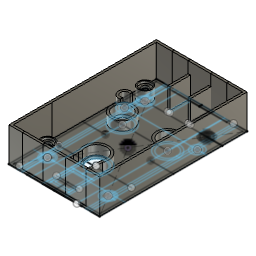
White_body v4 (Autodesk Fusion 360 design; units mm, degrees)
Autodesk Fusion 360 part; units mm, degrees
sketch "Sketch1" plane through (0, 0, 0) normal (0, 0, 1) x (1, 0, 0)
  line L0 (20, 32.5) -> (-20, 32.5)
  line L1 (-20, 32.5) -> (-20, -32.5)
  line L2 (-20, -32.5) -> (20, -32.5)
  line L3 (20, -32.5) -> (20, 32.5)
  line L4 (20, 32.5) -> (-20, -32.5) construction
  line L5 (-20, 32.5) -> (20, -32.5) construction
  line L6 (0, -32.5) -> (-5, -32.5)
  line L7 (-5, -32.5) -> (5, -32.5)
  line L8 (5, -32.5) -> (5, -16.2913)
  line L9 (-3.9274, -31.5) -> (4, -31.5)
  line L10 (-4, -17.7749) -> (-3.9274, -31.5)
  line L11 (4, -31.5) -> (4, -17.7749)
  line L12 (-5, -32.5) -> (-5, -16.2913)
  line L13 (-5, -16.2913) -> (-5, -32.5)
  line L14 (0, -31.5) -> (0, -32.5)
  circle A0 centre (0, -14) radius 4
  line L15 (4, -17.7749) -> (4, -16.0616)
  line L16 (19, -31.5) -> (19, 31.5)
  line L17 (19, 31.5) -> (-19, 31.5)
  line L18 (-19, 31.5) -> (-19, -31.5)
  line L19 (-19, -31.5) -> (19, -31.5)
  line L20 (-4, -17.7749) -> (-4, -16.0616)
  arc A1 (5, -16.2913) -> (-5, -16.2913) centre (0, -14) ccw
  arc A2 (4, -16.0616) -> (-4, -16.0616) centre (0, -14) ccw
  line L21 (-19, -30.875) -> (-17, -30.875)
  line L22 (-20, 32.5) -> (-14, 32.5)
  line L23 (-14, -32.5) -> (-14, 32.5)
  line L24 (-14, 32.5) -> (-14, 21.5)
  line L25 (-14, 21.5) -> (-20, 21.5)
  line L26 (-14, 21.5) -> (20, 21.5)
  line L27 (20, 21.5) -> (13.2308, 21.5)
  line L28 (14.03, -32.5) -> (14.03, 32.5)
  line L29 (-14, -32.5) -> (-14, -21.5)
  line L30 (-20, -21.5) -> (20, -21.5)
  circle A3 centre (-14, 21.5) radius 3
  circle A4 centre (13.2308, 21.5) radius 3
  circle A5 centre (-14, -21.5) radius 3
  circle A6 centre (14.03, -22.7988) radius 3
  line L31 (20, 21.5) -> (10.2308, 21.5)
  line L32 (20, 0) -> (10, 0)
  line L33 (10, 32.5) -> (10, -32.5)
  line L34 (-20, 0) -> (-10, 0)
  line L35 (-10, 32.5) -> (-10, -32.5)
  line L36 (10, 32.5) -> (10, 7.5)
  line L37 (10, 7.5) -> (-14, 7.5)
  circle A7 centre (-10, 7.5) radius 5
  circle A8 centre (10, 7.5) radius 5
  circle A9 centre (-10, 7.5) radius 4
  circle A10 centre (10, 7.5) radius 4
  line L38 (0, -32.5) -> (0, -27.5)
  line L39 (0, -27.5) -> (-5, -27.5)
  line L40 (5, -27.5) -> (0, -27.5)
  line L41 (0, -18) -> (0, -20)
  line L42 (0, -20) -> (-5, -20)
  line L43 (5, -20) -> (0, -20)
  line L44 (-3.9882, -20) -> (4.0118, -20)
  line L45 (4.0118, -20) -> (4.0118, -30)
  line L46 (4.0118, -30) -> (-3.9882, -30)
  line L47 (-3.9882, -30) -> (-3.9882, -20)
  line L48 (5, -26.5) -> (0, -26.5)
  line L49 (0, -26.5) -> (-5, -26.5)
  line L50 (-2.9882, -29) -> (-2.9882, -21)
  line L51 (-2.9882, -21) -> (3.0118, -21)
  line L52 (3.0118, -21) -> (3.0118, -29)
  line L53 (3.0118, -29) -> (-2.9882, -29)
  circle A11 centre (13.2308, 21.5) radius 2.5
  circle A12 centre (-14, 21.5) radius 2.5
  circle A13 centre (-14, -21.5) radius 2.5
  circle A14 centre (14.03, -22.7988) radius 2.5
  circle A15 centre (13.2308, 21.5) radius 2
  circle A16 centre (14.03, -22.7988) radius 2
  circle A17 centre (-14, -21.5) radius 2
  circle A18 centre (-14, 21.5) radius 2
  line L54 (20, -32.5) -> (16.0795, -32.5)
  line L55 (16.0795, -32.5) -> (16.0795, 32.5)
  line L56 (-20, 32.5) -> (-16, 32.5)
  line L57 (-16, 32.5) -> (-16, -32.5)
  line L58 (-16, -32.5) -> (-16, -14.5)
  line L59 (-16, -14.5) -> (16.0795, -14.5)
  line L60 (0, 32.5) -> (-5, 32.5)
  line L61 (-5, 32.5) -> (-5, 22.5)
  line L62 (0, 31.5) -> (0, 32.5)
  line L63 (0, 32.5) -> (5, 32.5)
  line L64 (5, 32.5) -> (5, 22.5)
  line L65 (0, 31.5) -> (0, 32.5)
  line L66 (0, 31.5) -> (-4, 31.5)
  line L67 (-4, 31.5) -> (-4, 22.5)
  line L68 (0, 31.5) -> (4, 31.5)
  line L69 (4, 31.5) -> (4, 22.5)
  line L70 (-16, 32.5) -> (-16, 14.5)
  line L71 (-20, 14.5) -> (20, 14.5)
  circle A19 centre (-16, 14.5) radius 2.75
  circle A20 centre (16.0795, 14.5) radius 2.75
  circle A21 centre (-16, 14.5) radius 1.75
  circle A22 centre (16.0795, 14.5) radius 1.75
  arc A23 (-19, -14.4988) -> (-19, -14.5012) centre (-16, -14.5) ccw
  arc A24 (19, -14.5012) -> (19, -14.4988) centre (16, -14.5) ccw
  line L72 (0, 31.5) -> (-12, 31.5)
  line L73 (-12, 31.5) -> (-12, 32.5)
  line L74 (-12, 32.5) -> (0, 32.5)
  line L75 (0, 32.5) -> (0, 31.5)
  line L76 (0, 31.5) -> (12, 31.5)
  line L77 (12, 31.5) -> (12, 32.5)
  line L78 (12, 32.5) -> (0, 32.5)
  line L79 (0, 32.5) -> (0, 31.5)
  line L80 (0, -32.5) -> (12, -32.5)
  line L81 (12, -32.5) -> (12, -31.5)
  line L82 (12, -31.5) -> (-12, -31.5)
  line L83 (-12, -31.5) -> (-12, -32.5)
  line L84 (-12, -32.5) -> (12, -32.5)
  line L85 (20, 32.5) -> (15, 32.5)
  line L86 (15, 32.5) -> (15, -32.5)
  line L87 (-20, -32.5) -> (-15, -32.5)
  line L88 (-15, -32.5) -> (-15.2402, 32.5)
  dimension "d1" = 40
  dimension "d2" = 65
  dimension "d4" = 10
  dimension "d13" = -1
  dimension "d16" = 11
  dimension "d18" = 11
  dimension "d19" = 6
  dimension "d20" = 6
  dimension "d21" = 6
  dimension "d22" = 6
  dimension "d23" = 10
  dimension "d25" = 10
  dimension "d26" = 25
  dimension "d27" = 10
  dimension "d28" = 10
  dimension "d29" = -1
  dimension "d30" = -1
  dimension "d31" = 5
  dimension "d32" = 8
  dimension "d33" = 10
  dimension "d34" = 1
  dimension "d35" = 1
  dimension "d36" = -0.5
  dimension "d37" = -0.5
  dimension "d38" = -0.5
  dimension "d39" = -0.5
  dimension "d40" = -1
  dimension "d41" = -1
  dimension "d42" = -1
  dimension "d43" = -1
  dimension "d44" = 18
  dimension "d45" = 6
  dimension "d50" = 5
  dimension "d52" = -1
  dimension "d53" = 1
  dimension "d54" = 18
  dimension "d55" = 5.5
  dimension "d56" = 5.5
  dimension "d57" = -1
  dimension "d58" = -1
  dimension "d59" = 12
  dimension "d60" = 12
  dimension "d61" = 24
  constraint horizontal L0
  constraint perpendicular L0 L1
  constraint parallel L0 L2
  constraint parallel L1 L3
  constraint coincident L4 origin
  constraint coincident L5 origin
  constraint perpendicular L6 L12
  constraint coincident L2 L6.end
  constraint parallel L2 L6
  constraint midpoint L2 L6.start
  constraint horizontal L7
  constraint vertical L8
  constraint parallel L11 L15
  constraint vertical L20
  constraint coincident L9 L14.start
  constraint coincident L4 L21.start
  constraint coincident L18 L21.start
  constraint perpendicular L18 L21
  constraint coincident L0 L22.end
  constraint coincident L2 L23.start
  constraint perpendicular L22 L23
  constraint perpendicular L17 L24
  constraint coincident L1 L25.end
  constraint perpendicular L1 L25
  constraint coincident L3 L26.end
  constraint perpendicular L3 L26
  constraint coincident L26 L27.end
  constraint coincident L4 L27.end
  constraint coincident L2 L28.start
  constraint perpendicular L0 L28
  constraint perpendicular L19 L29
  constraint coincident L1 L30.start
  constraint coincident L3 L30.end
  constraint perpendicular L3 L30
  constraint coincident L24.end L25.start
  constraint coincident L27.end A4.centre
  constraint coincident L29.end A5.centre
  constraint coincident L5 A6.centre
  constraint coincident L28 A6.centre
  constraint coincident L26 L31.end
  constraint coincident A4 L31.end
  constraint midpoint L3 L32.start
  constraint perpendicular L16 L32
  constraint coincident L0 L33.start
  constraint perpendicular L2 L33
  constraint midpoint L1 L34.start
  constraint perpendicular L23 L34
  constraint coincident L0 L35.start
  constraint coincident L2 L35.end
  constraint perpendicular L2 L35
  constraint parallel L33 L36
  constraint coincident L23 L37.end
  constraint perpendicular L23 L37
  constraint coincident L37 A7.centre
  constraint coincident L35 A7.centre
  constraint coincident L36.end L37.start
  constraint perpendicular L9 L38
  constraint coincident L13 L39.end
  constraint perpendicular L13 L39
  constraint coincident L8 L40.start
  constraint perpendicular L38 L40
  constraint coincident A0 L41.start
  constraint vertical L41
  constraint coincident L12 L42.end
  constraint perpendicular L12 L42
  constraint coincident L8 L43.start
  constraint perpendicular L41 L43
  constraint horizontal L44
  constraint vertical L45
  constraint horizontal L46
  constraint vertical L47
  constraint coincident L10 L44.start
  constraint coincident L42 L44.start
  constraint coincident L2 L54.end
  constraint coincident L0 L55.end
  constraint perpendicular L0 L55
  constraint coincident L0 L56.end
  constraint coincident L2 L57.end
  constraint perpendicular L2 L57
  constraint parallel L57 L58
  constraint coincident L55 L59.end
  constraint perpendicular L55 L59
  constraint coincident L58.end L59.start
  constraint perpendicular L60 L61
  constraint parallel L61 L62
  constraint coincident L0 L60.end
  constraint perpendicular L57 L60
  constraint midpoint L0 L60.start
  constraint horizontal L63
  constraint vertical L64
  constraint vertical L65
  constraint coincident L17 L62.start
  constraint perpendicular L56 L70
  constraint coincident L1 L71.start
  constraint coincident L3 L71.end
  constraint perpendicular L3 L71
  constraint coincident L70.end A19.centre
  constraint coincident L71 A20.centre
  constraint coincident L55 A20.centre
  constraint coincident L18 A23.start
  constraint coincident L18 A23.end
  constraint coincident L16 A24.end
  constraint coincident L16 A24.start
  constraint perpendicular L72 L73
  constraint parallel L72 L74
  constraint parallel L73 L75
  constraint perpendicular L35 L72
  constraint perpendicular L76 L77
  constraint parallel L76 L78
  constraint parallel L77 L79
  constraint perpendicular L28 L76
  constraint perpendicular L8 L80
  constraint coincident L19 L81.end
  constraint perpendicular L19 L81
  constraint perpendicular L35 L82
  constraint coincident L2 L83.end
  constraint perpendicular L2 L83
  constraint coincident L0 L85.end
  constraint coincident L2 L86.end
  constraint perpendicular L2 L86
  constraint coincident L2 L87.end
  constraint coincident L0 L88.end
  measures "d1" distance of L1.end L2.end
  measures "d2" distance of L0.end L1.end
  measures "d4" distance of L6.end L7.end
  measures "d16" distance of L22.end L24.end
  measures "d18" distance of L23.start L29.end
  measures "d19" diameter of A3
  measures "d20" diameter of A4
  measures "d21" diameter of A5
  measures "d22" diameter of A6
  measures "d23" distance of L32.start L32.end
  measures "d25" distance of L34.start L34.end
  measures "d26" distance of L33.start L36.end
  measures "d27" diameter of A7
  measures "d28" diameter of A8
  measures "d31" distance of L6.start L38.end
  measures "d32" distance of L44.start L44.end
  measures "d33" distance of L44.start L46.end
  measures "d44" distance of L57.end L58.end
  measures "d45" diameter of A23
  measures "d50" distance of L60.start L63.end
  measures "d54" distance of L56.end L70.end
  measures "d55" diameter of A19
  measures "d56" diameter of A20
  measures "d59" distance of L62.start L76.end
  measures "d60" distance of L6.start L80.end
  measures "d61" distance of L81.end L82.end
extrude "Extrude3" add sketch "Sketch1" along normal blind 15 contours L0 L3 L16 L17 L26 L27 L31 L55 L85 | L0 L17 L55 L85 L86 | L3 L16 L26 L27 L31 L71 | L0 L17 L28 L86 | L3 L16 L32 L71 | L0 L17 L28 L77 | L3 L16 L30 L32 A24 | L2 L3 L16 L19 L30 L54 L55 | L0 L17 L62 L63 L64 L65 L68 L75 L76 L78 L79 | L2 L19 L55 L86 | L0 L17 L60 L61 L62 L65 L66 L72 L74 L75 L79 | L2 L19 L28 L86 | L0 L17 L23 L24 L73 | L0 L17 L22 L23 L24 L88 | L2 L7 L8 L9 L14 L19 L38 L80 L82 L84 | L0 L17 L22 L57 L70 L88 | L2 L6 L7 L9 L12 L13 L14 L19 L38 L82 L84 | L0 L1 L17 L18 L22 L25 L56 L57 L70 | L1 L18 L25 L71 | L1 L18 L34 L71 | L1 L18 L30 L34 A23 | L2 L19 L23 L29 L88 | L1 L2 L18 L19 L30 L57 L58 L87 | L2 L19 L57 L58 L87 L88 makes body 1 at (20, -10.8333, 5) makes body 2 at (-20, 10.8333, 5) makes body 3 at (1.6667, 32.5, 5) makes body 4 at (-1.6667, -32.5, 5)
extrude "Extrude4" add sketch "Sketch1" along normal blind 5 contours L28 A8 | L28 L33 L36 A8 A10 | L33 L36 L37 A8 A10 | L33 L37 A8 A10 | L35 L37 A7 A9 | L23 L35 A7 A9 | A1 A2 L59 | L8 L11 L15 A1 A2 L43 L44 L59 | L35 L37 A7 A9 | L23 A7 | L8 L30 L43 L45 | L8 L30 L45 L48 | L10 L12 L13 L20 A1 A2 L42 L59 | L23 L35 A7 A9 | L8 L11 L19 L40 L45 L46 L82 | L8 L40 L45 L48 | L12 L13 L30 L42 L47 | L10 L12 L13 L19 L39 L46 L47 L82 | L12 L13 L30 L47 L49 | L12 L13 L39 L47 L49 bodies 4 makes body 5 at (-5.0248, 7.9978, 3.3333) makes body 6 at (14.9752, 7.0022, 1.6667)
sketch "Sketch2" plane through (0, 0, 0) normal (0, 0, 1) x (1, 0, 0)
  line L0 (5.0501, 21.5139) -> (-4.9499, 21.5139)
  line L1 (5.0501, 22.5139) -> (-4.9499, 22.5139)
  line L2 (-4.9499, 21.5139) -> (5.0501, 21.5139)
  line L3 (5.0501, 21.5139) -> (5.0501, 32.5139)
  line L4 (5.0501, 32.5139) -> (-4.9499, 32.5139)
  line L5 (-4.9499, 32.5139) -> (-4.9499, 21.5139)
  line L6 (-3.9499, 22.5139) -> (4.0501, 22.5139)
  line L7 (4.0501, 22.5139) -> (4.0501, 31.5139)
  line L8 (4.0501, 31.5139) -> (-3.9499, 31.5139)
  line L9 (-3.9499, 31.5139) -> (-3.9499, 22.5139)
  line L10 (-4.9499, 22.5139) -> (5.0501, 22.5139)
  dimension "d66" = 10
  dimension "d67" = 1
  dimension "d68" = 10
  dimension "d69" = 11
  dimension "d70" = -1
  constraint horizontal L0
  constraint horizontal L2
  constraint vertical L3
  constraint horizontal L4
  constraint vertical L5
  measures "d66" distance of L0.start L0.end
  measures "d68" distance of L0.end L0.start
  measures "d69" distance of L0.end L4.end
extrude "Extrude5" add sketch "Sketch2" along normal blind 10 contours L1 L3 L4 L5 L7 L8 L9 L10 bodies 3
extrude "Extrude6" add sketch "Sketch1" along normal blind 6 separate body contours L26 L27 A4 L31 A11 L55 L86 | L26 L27 A4 L31 L55 | L26 L27 A4 L31 L55 | L28 A4 A11 L86 | L26 L27 A4 L31 A11 L55 L86 | L26 L28 A4 L31 A11 | L28 A4 A11 L86 | L26 L28 A4 L31 A11 | L30 A6 A14 L55 | L30 A6 A14 L55 | A6 A14 L55 L86 | A6 A14 L55 L86 | L28 A6 A14 L86 | L23 L26 A3 A12 | L23 L24 L26 A3 A12 | L28 A6 A14 L86 | L28 L30 A6 A14 | L23 L24 A3 A12 L88 | L23 A3 A12 L88 | L28 L30 A6 A14 | A3 A12 L57 L70 L88 | A3 A12 L57 L70 L88 | L25 A3 A12 L57 L70 | L25 A3 A12 L57 L70 | L23 L29 L30 A5 A13 | L23 L30 A5 A13 | L23 A5 A13 L88 | A5 A13 L57 L58 L88 | L23 L29 A5 A13 L88 | L30 A5 A13 L57 L58 | A5 A13 L57 L58 L88 | L30 A5 A13 L57 L58 makes body 7 at (16.2159, 21.7987, 4) makes body 8 at (-11.0149, -21.2013, 4) makes body 9 at (-11.0149, 21.2013, 2) makes body 10 at (17.0151, -22.5001, 4)
extrude "Extrude7" add sketch "Sketch1" along normal blind 5 contours L28 A11 A15 L86 | L26 L27 L31 A11 A15 L86 | L26 L27 L31 A11 A15 L86 | L26 L28 L31 A11 A15 | L28 A11 A15 L86 | L26 L28 L31 A11 A15 | L30 A14 L55 | L30 A14 L55 | L30 A14 A16 L55 L86 | L30 A14 A16 L55 L86 | L28 A14 A16 L86 | L23 L26 A12 A18 | L23 L24 L26 A12 A18 | L28 A14 A16 L86 | L28 L30 A14 A16 | L23 L24 A12 A18 L88 | L23 A12 A18 L88 | L28 L30 A14 A16 | A12 A18 L57 L70 L88 | A12 A18 L57 L70 L88 | L25 A12 L57 L70 | L25 A12 L57 L70 | L23 L29 L30 A13 A17 | L23 L30 A13 A17 | L23 A13 A17 L88 | A13 A17 L57 L58 L88 | L23 L29 A13 A17 L88 | L30 A13 L57 L58 | A13 A17 L57 L58 L88 | L30 A13 L57 L58 bodies 7 8 9 10
extrude "Extrude8" add sketch "Sketch1" 10 faces at (15.8788, 21.2516, 0) (-4.6627, -22.9304, 0) (-11.3519, -21.7484, 0) (16.6855, -22.9479, 0) (-19.6667, -4.8335, 0) (14.6332, 7.0529, 0) (19.6667, -4.8332, 0) (-11.3519, 21.2516, 0) (-5.3519, 7.2516, 0) (-1.2833, 32.1759, 0) along normal blind 1 contours L0 L3 L16 L17 L26 L27 L31 L55 L85 | L0 L17 L55 L85 L86 | L3 L16 L26 L27 L31 L71 | L0 L17 L28 L86 | L17 A4 L55 L86 | L16 L17 L26 L27 A4 L31 L55 | L3 L16 L32 L71 | L16 L26 L27 A4 L31 L55 L71 A20 | L0 L17 L28 L77 | L17 L28 A4 L86 | L26 L27 A4 L31 A11 L55 L86 | L26 L27 A4 L31 L55 | L3 L16 L30 L32 A24 | L16 L32 L55 L71 A20 | L26 L27 A4 L31 L55 | L17 L26 L28 A4 L33 L36 L76 | L28 A4 A11 L86 | L26 L27 A4 L31 A11 L55 L86 | L2 L3 L16 L19 L30 L54 L55 | L16 L30 A6 L32 L55 A24 | L55 L71 A20 A22 | L55 L71 A20 A22 | A4 L55 A20 L86 | L26 L28 A4 L31 A11 | L28 A11 A15 L86 | L26 L27 L31 A11 A15 L86 | L26 L27 L31 A11 A15 L86 | L16 L19 L30 A6 L55 | L32 L55 L59 L86 | L32 L55 A20 L86 | L55 L71 A22 | L55 L71 A22 | L55 A20 A22 L86 | L55 A20 A22 L86 | L28 A4 A20 L86 | L28 A4 A11 L86 | L0 L17 L62 L63 L64 L65 L68 L75 L76 L78 L79 | L17 L26 L33 L35 L36 L66 L68 L72 L76 | L26 L28 L31 A11 A15 | L26 L28 A4 L33 L36 L71 A20 | L26 L28 A4 L31 A11 | L26 L27 L28 L31 A15 L86 | L26 L27 L31 A15 L86 | L26 L27 L31 A15 L86 | L28 A11 A15 L86 | L2 L19 L55 L86 | L30 A6 A14 L55 | L30 A6 A14 L55 | L28 L32 L59 L86 | L28 L32 A8 L86 | A6 L55 L59 L86 | L55 L71 A22 L86 | L55 L71 A22 L86 | L28 L71 A20 A22 L86 | L28 A8 A20 L86 | L28 L71 A20 A22 L86 | L0 L17 L60 L61 L62 L65 L66 L72 L74 L75 L79 | L26 L33 L35 L36 L71 | L26 L27 L28 L31 A15 | L26 L28 L31 A11 A15 | L26 L27 L28 L31 A15 L86 | L2 L19 L28 L86 | L19 A6 L55 L86 | L30 A14 L55 | L30 A14 L55 | A6 A14 L55 L86 | L28 L32 L33 A8 | L28 L32 L33 L59 | L28 A8 | L28 A6 L59 L86 | L71 A22 L86 | L71 A22 L86 | L28 L71 A20 | L28 L71 A20 | L28 L33 L36 A8 L71 A20 | L23 L26 A3 L35 L71 A19 | L17 L23 L24 L26 A3 L35 L72 | L33 L35 L36 L37 A7 A8 L71 | L26 L27 L28 L31 A15 | L19 L28 A6 L86 | A6 A14 L55 L86 | L30 A14 A16 L55 L86 | L30 A14 A16 L55 L86 | L28 A6 A14 L86 | L28 L30 A6 L33 L59 | L28 L33 L36 A8 A10 | A1 L33 L35 L37 A7 A8 L59 | L23 L26 A3 A12 | L23 L24 L26 A3 A12 | L23 L35 A7 L71 A19 | L33 L36 L37 A8 A10 | L19 L28 L30 A6 L33 L82 | L28 A6 A14 L86 | L30 A16 L86 | L30 A16 L86 | L28 A14 A16 L86 | L28 L30 A6 A14 | L8 A1 L30 L33 L59 | L33 L37 A8 A10 | L0 L17 L23 L24 L73 | L23 L26 A12 A18 | L23 L24 L26 A12 A18 | L17 L23 L24 A3 L88 | L23 L24 A3 A12 L88 | L23 A3 A12 L88 | L23 A3 A19 L88 | L35 L37 A7 A9 | L23 L35 A7 A9 | L23 L71 A19 | L23 L71 A19 | L28 L30 A6 A14 | L28 A14 A16 L86 | L28 L30 A16 L86 | L28 L30 A16 L86 | L28 L30 A14 A16 | L8 L19 L30 L33 L82 | A1 A2 L59 | L8 L11 L15 A1 A2 L43 L44 L59 | L0 L17 L22 L23 L24 L88 | L23 L26 A18 | L23 L24 L26 A18 | L23 L24 A12 A18 L88 | L23 A12 A18 L88 | A3 A12 L57 L70 L88 | L17 A3 L57 L70 L88 | L23 L71 A19 A21 L88 | A3 L57 L70 A19 L88 | A3 A12 L57 L70 L88 | L35 L37 A7 A9 | L23 L34 A7 A19 L88 | L23 A7 | L23 L71 A19 A21 L88 | L2 L7 L8 L9 L14 L19 L38 L80 L82 L84 | L28 L30 A14 A16 | L28 L30 A16 | L28 L30 A16 | L8 L30 L43 L45 | L8 L30 L45 L48 | L10 L12 L13 L20 A1 A2 L42 L59 | L12 L13 A1 L30 L35 L59 | A0 A2 L59 | L11 A0 L15 A2 L41 L43 L44 L59 | L0 L17 L22 L57 L70 L88 | L23 L24 L25 A18 L88 | L23 L25 A18 L88 | A12 A18 L57 L70 L88 | A12 A18 L57 L70 L88 | L25 A3 A12 L57 L70 | L17 L18 L25 A3 L57 L70 | L57 L70 A19 A21 L88 | L18 L25 A3 L57 L70 L71 A19 | L25 A3 A12 L57 L70 | L23 L35 A7 A9 | L23 L34 L35 A7 | L71 A21 L88 | L71 A21 L88 | L34 L57 A19 L88 | L57 A19 A21 L88 | L2 L6 L7 L9 L12 L13 L14 L19 L38 L82 L84 | L8 L11 L19 L40 L45 L46 L82 | L8 L40 L45 L48 | L11 L30 L45 L48 | L11 L30 L43 L44 L45 | L23 L34 L35 L59 | L23 L30 A5 L35 L59 | L10 A0 L20 A2 L41 L42 L44 L59 | L0 L1 L17 L18 L22 L25 L56 L57 L70 | L25 A18 L88 | L25 A18 L88 | L25 A12 L57 L70 | L25 A12 L57 L70 | L57 L70 L71 A19 A21 | L57 L70 L71 A21 L88 | L23 L34 L59 L88 | L57 L71 A21 L88 | L57 L71 A19 A21 | L18 L34 L57 L71 A19 | L34 L57 L59 L88 | L9 L11 L19 L38 L46 L82 | L9 L10 L19 L38 L46 L82 | L11 L40 L45 L48 | L10 L11 L30 L42 L43 L44 L50 L51 L52 | L11 L30 L48 L52 | L12 L13 L30 L42 L47 | L19 L23 L29 L30 A5 L35 L82 | L12 L13 L19 L30 L35 L82 | L23 A5 L59 L88 | L1 L18 L25 L71 | L57 L70 L71 A21 | L57 L71 A21 | L18 L30 A5 L34 L57 L58 A23 | A5 L57 L58 L59 L88 | L10 L12 L13 L19 L39 L46 L47 L82 | L10 L38 L39 L46 L50 L53 | L11 L38 L40 L46 L52 L53 | L11 L40 L45 L46 | L11 L40 L48 L52 | L12 L13 L30 L47 L49 | L10 L30 L47 | L23 L29 L30 A5 A13 | L23 L30 A5 A13 | L23 A5 A13 L88 | L1 L18 L34 L71 | L1 L18 L30 L34 A23 | A5 A13 L57 L58 L88 | L12 L13 L39 L47 L49 | L10 L39 L46 L47 | L10 L30 L49 L50 | L10 L30 L47 L49 | L23 L29 L30 A13 A17 | L23 L30 A13 A17 | L23 L29 A5 A13 L88 | L19 L23 L29 A5 L88 | L23 A13 A17 L88 | L30 A5 A13 L57 L58 | A13 A17 L57 L58 L88 | L2 L19 L23 L29 L88 | L10 L39 L47 L49 | L10 L39 L49 L50 | L23 L29 L30 A17 | L23 L30 A17 | L23 L29 A13 A17 L88 | L19 A5 L57 L58 L88 | A5 A13 L57 L58 L88 | L23 L30 A17 L88 | L1 L2 L18 L19 L30 L57 L58 L87 | L18 L19 L30 A5 L57 L58 | L30 A5 A13 L57 L58 | L30 A13 L57 L58 | L30 A17 L88 | L2 L19 L57 L58 L87 L88 | L23 L29 L30 A17 L88 | A13 A17 L57 L58 L88 | L30 A13 L57 L58 | L30 A17 L88 on bodies 1 2 3 4 5 6 7 8 9 10 bodies 7 1 2 3 4 5 6 8 9 10
extrude "Extrude9" add sketch "Sketch1" along normal blind 1 contours L0 L17 L33 L36 L76 L77 L78 | L0 L17 L33 L36 L64 L76 L78 | L0 L17 L35 L61 L72 L74 | L2 L19 L28 L81 | L0 L17 L35 L72 L73 L74 | L2 L19 L33 L80 L81 L82 L84 | L2 L8 L19 L33 L80 L82 L84 | L2 L12 L13 L19 L35 L82 L84 | L2 L19 L35 L82 L83 L84 | L2 L19 L23 L29 L83 bodies 7
extrude "Extrude10" add sketch "Sketch1" along normal blind 5 contours L55 L71 A20 A22 | L55 L71 A20 A22 | L55 A20 A22 L86 | L55 A20 A22 L86 | L57 L70 A19 A21 L88 | L57 A19 A21 L88 | L57 L70 L71 A19 A21 | L57 L71 A19 A21 bodies 7
extrude "Extrude11" add sketch "Sketch1" along normal blind 5 contours L26 L27 L28 L31 A15 L86 | L26 L27 L31 A15 L86 | L26 L27 L31 A15 L86 | L26 L27 L28 L31 A15 | L26 L27 L28 L31 A15 L86 | L26 L27 L28 L31 A15 | L30 A16 L86 | L30 A16 L86 | L28 L30 A16 L86 | L28 L30 A16 L86 | L23 L26 A18 | L23 L24 L26 A18 | L28 L30 A16 | L28 L30 A16 | L23 L24 L25 A18 L88 | L23 L25 A18 L88 | L25 A18 L88 | L25 A18 L88 | L23 L29 L30 A17 | L23 L30 A17 | L23 L30 A17 L88 | L30 A17 L88 | L23 L29 L30 A17 L88 | L30 A17 L88 bodies 7
hole "Hole1" at (-14, 21.5, 5) direction (0, 0, -1) diameter 2.18 depth 4 tip angle 118 counterbore diameter 3 counterbore depth 1 bodies 7
thread "Thread1" "ISO Metric profile 2.6 M2.6x0.45 6H"
hole "Hole2" at (13.2308, 21.5, 5) direction (0, 0, -1) diameter 2.18 depth 4 tip angle 118 counterbore diameter 3 counterbore depth 1 bodies 7
thread "Thread2" "ISO Metric profile 2.6 M2.6x0.45 6H"
hole "Hole3" at (14.03, -22.7988, 5) direction (0, 0, -1) diameter 2.18 depth 4 tip angle 118 counterbore diameter 3 counterbore depth 1 bodies 7
thread "Thread3" "ISO Metric profile 2.6 M2.6x0.45 6H"
hole "Hole4" at (-14, -21.5, 5) direction (0, 0, -1) diameter 2.18 depth 4 tip angle 118 counterbore diameter 3 counterbore depth 1 bodies 7
thread "Thread4" "ISO Metric profile 2.6 M2.6x0.45 6H"
extrude "Extrude1" add sketch "Sketch1" along normal blind 1 separate body makes body 11
extrude "Extrude2" add sketch "Sketch1" along normal blind 15 contours L0 L3 L16 L17 L26 L27 L31 L55 L85 | L0 L17 L55 L85 L86 | L3 L16 L26 L27 L31 L71 | L0 L17 L28 L86 | L3 L16 L32 L71 | L0 L17 L28 L77 | L3 L16 L30 L32 A24 | L0 L17 L33 L36 L76 L77 L78 | L2 L3 L16 L19 L30 L54 L55 | L0 L17 L33 L36 L64 L76 L78 | L0 L17 L62 L63 L64 L65 L68 L75 L76 L78 L79 | L2 L19 L55 L86 | L0 L17 L60 L61 L62 L65 L66 L72 L74 L75 L79 | L2 L19 L28 L86 | L0 L17 L35 L61 L72 L74 | L2 L19 L28 L81 | L0 L17 L35 L72 L73 L74 | L2 L19 L33 L80 L81 L82 L84 | L0 L17 L23 L24 L73 | L2 L8 L19 L33 L80 L82 L84 | L0 L17 L22 L23 L24 L88 | L2 L7 L8 L9 L14 L19 L38 L80 L82 L84 | L0 L17 L22 L57 L70 L88 | L2 L6 L7 L9 L12 L13 L14 L19 L38 L82 L84 | L0 L1 L17 L18 L22 L25 L56 L57 L70 | L2 L12 L13 L19 L35 L82 L84 | L1 L18 L25 L71 | L2 L19 L35 L82 L83 L84 | L1 L18 L34 L71 | L1 L18 L30 L34 A23 | L2 L19 L23 L29 L83 | L2 L19 L23 L29 L88 | L1 L2 L18 L19 L30 L57 L58 L87 | L2 L19 L57 L58 L87 L88 bodies 11
extrude "Extrude12" cut sketch "Sketch1" along normal blind 1 contours L33 L36 A10 | L33 L36 L37 A10 | L33 L37 A10 | L35 L37 A9 | L35 L37 A9 | L35 L37 A9 | L35 L37 A9 | A0 L59 | A0 L59 bodies 11
extrude "Extrude13" cut sketch "Sketch1" along normal blind 1 contours L30 L48 L49 L50 L52 | L30 L50 L51 L52 | L38 L39 L50 L53 | L38 L40 L52 L53 | L39 L40 L48 L49 L50 L52 bodies 11
